Autodesk Inventor part; units mm, degrees
(part 2 of 2)
sketch "Sketch24" plane through (0, 0, 0) normal (0, -1, 0) x (1, 0, 0)
  line L0 (-11.769848, -363.559848) -> (-207.349848, -363.559848)
  line L1 (-109.559848, -363.559848) -> (-77.809848, -363.559848)
  line L2 (-77.809848, -363.559848) -> (-77.809848, -325.459848)
  line L3 (-77.809848, -325.459848) -> (-77.809848, -249.259848)
  line L4 (-77.809848, -325.459848) -> (-67.649848, -325.459848)
  line L5 (-67.649848, -325.459848) -> (-87.969848, -325.459848)
  line L6 (-77.809848, -249.259848) -> (-67.649848, -249.259848)
  line L7 (-67.649848, -249.259848) -> (-87.969848, -249.259848)
  line L8 (-109.559848, -363.559848) -> (-141.309848, -363.559848)
  line L9 (-141.309848, -363.559848) -> (-141.309848, -325.459848)
  line L10 (-141.309848, -325.459848) -> (-141.309848, -249.259848)
  line L11 (-141.309848, -325.459848) -> (-131.149848, -325.459848)
  line L12 (-131.149848, -325.459848) -> (-151.469848, -325.459848)
  line L13 (-141.309848, -249.259848) -> (-131.149848, -249.259848)
  line L14 (-131.149848, -249.259848) -> (-151.469848, -249.259848)
  circle A0 centre (-67.649848, -249.259848) radius 1.778
  circle A1 centre (-87.969848, -249.259848) radius 1.778
  circle A2 centre (-67.649848, -325.459848) radius 1.778
  circle A3 centre (-87.969848, -325.459848) radius 1.778
  circle A4 centre (-131.149848, -325.459848) radius 1.778
  circle A5 centre (-151.469848, -325.459848) radius 1.778
  circle A6 centre (-131.149848, -249.259848) radius 1.778
  circle A7 centre (-151.469848, -249.259848) radius 1.778
  point P0 (0, 0)
  dimension "d150" = 31.75
  dimension "d151" = 38.1
  dimension "d152" = 76.2
  dimension "d153" = 10.16
  dimension "d154" = 20.32
  dimension "d155" = 10.16
  dimension "d156" = 20.32
  dimension "d157" = 31.75
  dimension "d158" = 38.1
  dimension "d159" = 76.2
  dimension "d160" = 10.16
  dimension "d161" = 20.32
  dimension "d162" = 10.16
  dimension "d163" = 20.32
  dimension "d164" = 3.556
  constraints: 28 end point, 8 centre point, 8 coincident, 5 perpendicular, 4 point on line, 3 collinear, 2 parallel, 1 midpoint
  measures "d150" distance of L1.start L1.end
  measures "d151" distance of L1.end L2.end
  measures "d152" distance of L2.end L3.end
  measures "d153" distance of L2.end L4.end
  measures "d154" distance of L4.end L5.end
  measures "d155" distance of L3.end L6.end
  measures "d156" distance of L6.end L7.end
  measures "d157" distance of L1.start L8.end
  measures "d158" distance of L8.end L9.end
  measures "d159" distance of L9.end L10.end
  measures "d160" distance of L9.end L11.end
  measures "d161" distance of L11.end L12.end
  measures "d162" distance of L10.end L13.end
  measures "d163" distance of L13.end L14.end
  measures "d164" diameter of A0
extrude "Extrusion23" cut sketch "Sketch24" against normal blind 6.35
body "Solid1"
